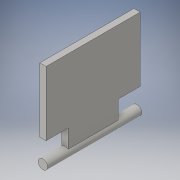
# Autodesk Inventor part: gpsDoor
Saved by Autodesk Inventor 2016 (Build 200138000, 138)
## iProperties
Created: 2016-10-13
Part Number: gpsDoor
Material: Generic
Document SubType Name: Modeling
Designer: lachesis
Density: 1 g/cm^3
Appearance: Default
Author: lachesis
Autodesk Inventor part; units mm, degrees
ref_plane "YZ Plane" through (0, 0, 0) normal (1, 0, 0) x (0, 1, 0)
ref_plane "XZ Plane" through (0, 0, 0) normal (0, 1, 0) x (-1, 0, 0)
ref_plane "XY Plane" through (0, 0, 0) normal (0, 0, 1) x (1, 0, 0)
sketch "Sketch1" plane through (0, 0, 0) normal (0, 0, 1) x (1, 0, 0)
  circle A0 centre (0, 0) radius 1.5
  dimension "d0" = 3
  constraints: 1 centre point, 1 coincident
  measures "d0" diameter of A0
extrude "Extrusion1" add sketch "Sketch1" along normal blind 30
ref_plane "Work Plane1" through (0, 0, 23) normal (0, 0, 1) x (1, 0, 0)
ref_plane "Work Plane2" through (0, 0, 7) normal (0, 0, -1) x (-1, 0, 0)
sketch "Sketch2" plane through (0, 0, 23) normal (0, 0, 1) x (1, 0, 0)
  circle A0 centre (0, 0) radius 1.5 projected
  line L0 (1, 0) -> (-1, 0)
  line L1 (-1, 0) -> (-1, 27.5)
  line L2 (-1, 27.5) -> (1, 27.5)
  line L3 (1, 27.5) -> (1, 0)
  dimension "d7" = 27.5
  dimension "d13" = 1
  constraints: 8 end point, 2 parallel, 1 coincident, 1 horizontal, 1 midpoint, 1 perpendicular
  measures "d7" distance from line of point (0, 0) L2
  measures "d13" distance from line of point (0, 0) L1
extrude "Extrusion2" add sketch "Sketch2" against normal up to surface (16 mm away) contours L3 L0 L1 A0 | A0 L1 L2 L3 picked at (0, 0.5)
sketch "Sketch3" plane through (1, 1.118, 23) normal (1, 0, 0) x (0, 0, -1)
  line L0 (16, 0) -> (16, 26.382) projected
  line L1 (0, 26.382) -> (16, 26.382) projected
  line L2 (0, 26.382) -> (0, 0) projected
  line L3 (16, 0) -> (0, 0) projected
  line L4 (0, 26.382) -> (-7, 26.382)
  line L5 (-7, 26.382) -> (-7, 5.882)
  line L6 (-7, 5.882) -> (0, 5.882)
  line L7 (0, 5.882) -> (0, 26.382)
  line L8 (16, 0) -> (16, 26.382) projected
  line L9 (16, 26.382) -> (23, 26.382)
  line L10 (23, 26.382) -> (23, 5.882)
  line L11 (23, 5.882) -> (16, 5.882)
  line L12 (16, 5.882) -> (16, 26.382)
  line L13 (23, -2.618) -> (23, 0.382) projected
  line L14 (-7, 0.382) -> (-7, -2.618) projected
  line L15 (0, 0) -> (16, 0) projected
  line L16 (16, 0) -> (16, 0) projected
  line L17 (16, 0) -> (0, 0) projected
  line L18 (0, 0) -> (0, 0) projected
  point P0 (23, -1.118)
  point P1 (19.5, 5.882)
  point P2 (-3.5, 5.882)
  point P3 (23, -1.118)
  point P4 (23, 16.132)
  point P5 (-7, 16.132)
  point P6 (-7, -1.118)
  dimension "d10" = 5.5
  constraints: 16 end point, 6 midpoint, 4 parallel, 2 horizontal, 2 perpendicular, 2 vertical alignment, 1 horizontal alignment
  measures "d10" distance from line of L13.end L11
extrude "Extrusion3" add sketch "Sketch3" against normal up to surface (2 mm away) contours L0 L9 L10 L11 | L6 L5 L4 L2
body "Solid1"
